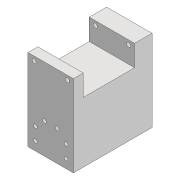
# Autodesk Inventor part: link
Saved by Autodesk Inventor 2020 (Build 240168000, 168)
## iProperties
Created: 2020-11-09
Part Number: link
Material: 일반
Document SubType Name: Modeling
Designer: 이호석
Mass: 68.2224 g
Surface Area: 145.151 cm^2
Volume: 68.2224 cm^3
Density: 1 g/cm^3
Appearance: 기본값
Author: 이호석
Autodesk Inventor part; units mm, degrees
ref_plane "YZ Plane" through (0, 0, 0) normal (1, 0, 0) x (0, 1, 0)
ref_plane "XZ Plane" through (0, 0, 0) normal (0, 1, 0) x (-1, 0, 0)
ref_plane "XY Plane" through (0, 0, 0) normal (0, 0, 1) x (1, 0, 0)
sketch "스케치1" plane through (0, 0, 0) normal (0, 0, 1) x (1, 0, 0)
  arc A0 (15, 100.5) -> (13, 102.5) centre (13, 100.5) ccw projected
  line L0 (13, 102.5) -> (-13, 102.5) projected
  arc A1 (-13, 102.5) -> (-15, 100.5) centre (-13, 100.5) ccw projected
  line L1 (-15, 100.5) -> (-15, -100.5) projected
  arc A2 (-15, -100.5) -> (-13, -102.5) centre (-13, -100.5) ccw projected
  line L2 (-13, -102.5) -> (-7, -102.5) projected
  arc A3 (-7, -102.5) -> (-5, -100.5) centre (-7, -100.5) ccw projected
  line L3 (-5, -100.5) -> (-5, -92.5) projected
  arc A4 (5, -92.5) -> (-5, -92.5) centre (0, -92.5) ccw projected
  line L4 (5, -92.5) -> (5, -100.5) projected
  arc A5 (5, -100.5) -> (7, -102.5) centre (7, -100.5) ccw projected
  line L5 (7, -102.5) -> (13, -102.5) projected
  arc A6 (13, -102.5) -> (15, -100.5) centre (13, -100.5) ccw projected
  line L6 (15, -100.5) -> (15, 100.5) projected
  circle A7 centre (7.7782, -100.2782) radius 1.25 projected
  circle A8 centre (0, -81.5) radius 1.25 projected
  circle A9 centre (-11, -92.5) radius 1.25 projected
  circle A10 centre (11, -92.5) radius 1.25 projected
  circle A11 centre (-7.7782, -100.2782) radius 1.25 projected
  circle A12 centre (7.7782, -84.7218) radius 1.25 projected
  circle A13 centre (-7.7782, -84.7218) radius 1.25 projected
  circle A14 centre (-10.1627, 76.7095) radius 1.25 projected
  circle A15 centre (-10.1627, 68.2905) radius 1.25 projected
  circle A16 centre (10.1627, 68.2905) radius 1.25 projected
  circle A17 centre (10.1627, 76.7095) radius 1.25 projected
  circle A18 centre (4.2095, 82.6627) radius 1.25 projected
  circle A19 centre (-4.2095, 82.6627) radius 1.25 projected
  line L7 (0, 102.5) -> (0, 82.5)
  line L8 (15, 102.5) -> (-15, 102.5)
  line L9 (-15, 102.5) -> (-15, 62.5)
  line L10 (-15, 62.5) -> (15, 62.5)
  line L11 (15, 62.5) -> (15, 102.5)
  line L12 (15, 102.5) -> (-15, 62.5) construction
  line L13 (-15, 102.5) -> (15, 62.5) construction
  point P0 (0, 0)
  dimension "d0" = 20
  dimension "d1" = 40
  constraints: 14 end point, 3 midpoint, 2 parallel, 1 horizontal, 1 perpendicular, 1 point on line, 1 vertical
  measures "d0" distance of L7.start L7.end
  measures "d1" distance of L9.end L8.end
ref_plane "작업 평면1" through (-15, -102.5, 52) normal (0, 0, -1) x (0, 1, 0)
extrude "돌출1" add sketch "스케치1" along normal up to surface (52 mm away) contours L6 L10 L1 A1 L0 A0
sketch "스케치2" plane through (-13, 102.5, 0) normal (0, 1, 0) x (1, 0, 0)
  line L0 (-0.4121, -11.5) -> (26.4121, -11.5) projected
  line L1 (-0.4121, -45.5) -> (26.4121, -45.5) projected
  line L2 (-2, 0) -> (-2, -52) projected
  line L3 (28, 0) -> (28, -52) projected
  line L4 (-2, -52) -> (28, -52)
  line L5 (28, -52) -> (28, -45.5)
  line L6 (28, -45.5) -> (-2, -45.5)
  line L7 (-2, -45.5) -> (-2, -52)
  line L8 (-2, 0) -> (28, 0)
  line L9 (28, 0) -> (28, -11.5)
  line L10 (28, -11.5) -> (-2, -11.5)
  line L11 (-2, -11.5) -> (-2, 0)
  point P0 (13, 0)
  dimension "d4" = 30
  constraints: 16 end point, 4 parallel, 3 point on line, 2 horizontal, 2 perpendicular
  measures "d4" distance of L9.end L10.end
ref_plane "작업 평면2" through (-7.15, 116.5, 9.5) normal (0, -1, 0) x (1, 0, 0)
extrude "돌출2" add sketch "스케치2" along normal up to surface (14 mm away) contours L10 L2 L8 L3 L0 | L6 L1 L3 L4 L2
sketch "스케치3" plane through (0, 0, 0) normal (0, 0, -1) x (-1, 0, 0)
  line L0 (-15, 102.5) -> (-13, 102.5) projected
  line L1 (-15, 62.5) -> (-15, 100.5) projected
  line L2 (-15, 102.5) -> (-15, 100.5)
  line L3 (15, 100.5) -> (15, 62.5) projected
  line L4 (-15, 100.5) -> (15, 100.5)
  line L5 (15, 100.5) -> (15, 102.5)
  arc A0 (15, 100.5) -> (13, 102.5) centre (13, 100.5) ccw projected
  line L6 (-15, 102.5) -> (15, 102.5)
  line L7 (13, 102.5) -> (-13, 102.5) projected
  point P0 (0, 0)
  constraints: 8 end point, 2 perpendicular, 1 collinear, 1 tangent, 1 vertical
extrude "돌출3" add sketch "스케치3" against normal up to surface (52 mm away)
sketch "스케치4" plane through (0, 0, 0) normal (0, 0, -1) x (-1, 0, 0)
  circle A0 centre (-17.3, 119) radius 1.35 projected
  circle A1 centre (17.3, 119) radius 1.35 projected
  line L0 (-20.1, 119.3234) -> (-20.1, 163.5766) projected
  arc A2 (-20.1, 119.3234) -> (-19.5808, 117.6364) centre (-17.1, 119.3234) ccw projected
  line L1 (-15.8929, 112.2131) -> (-19.5808, 117.6364) projected
  arc A3 (-15.8929, 112.2131) -> (-13.4121, 110.9) centre (-13.4121, 113.9) ccw projected
  line L2 (13.4121, 110.9) -> (-13.4121, 110.9) projected
  arc A4 (13.4121, 110.9) -> (15.8929, 112.2131) centre (13.4121, 113.9) ccw projected
  line L3 (19.5808, 117.6364) -> (15.8929, 112.2131) projected
  arc A5 (19.5808, 117.6364) -> (20.1, 119.3234) centre (17.1, 119.3234) ccw projected
  line L4 (20.1, 163.5766) -> (20.1, 119.3234) projected
  arc A6 (20.1, 163.5766) -> (19.5808, 165.2636) centre (17.1, 163.5766) ccw projected
  line L5 (15.5953, 171.1246) -> (19.5808, 165.2636) projected
  arc A7 (15.5953, 171.1246) -> (13.9414, 172) centre (13.9414, 170) ccw projected
  line L6 (6.65, 172) -> (13.9414, 172) projected
  arc A8 (8.15, 170.5) -> (6.65, 172) centre (6.65, 170.5) ccw projected
  line L7 (8.15, 170.5) -> (8.15, 168) projected
  arc A9 (8.15, 168) -> (10.5, 165.65) centre (10.5, 168) ccw projected
  line L8 (10.5, 165.65) -> (13.5, 165.65) projected
  arc A10 (14.5, 164.65) -> (13.5, 165.65) centre (13.5, 164.65) ccw projected
  line L9 (14.5, 164.65) -> (14.5, 123.85) projected
  arc A11 (13.5, 122.85) -> (14.5, 123.85) centre (13.5, 123.85) ccw projected
  line L10 (13.5, 122.85) -> (10.5, 122.85) projected
  arc A12 (10.5, 122.85) -> (8.15, 120.5) centre (10.5, 120.5) ccw projected
  line L11 (8.15, 120.5) -> (8.15, 117.5) projected
  arc A13 (7.15, 116.5) -> (8.15, 117.5) centre (7.15, 117.5) ccw projected
  line L12 (7.15, 116.5) -> (-7.15, 116.5) projected
  arc A14 (-8.15, 117.5) -> (-7.15, 116.5) centre (-7.15, 117.5) ccw projected
  line L13 (-8.15, 117.5) -> (-8.15, 120.5) projected
  arc A15 (-8.15, 120.5) -> (-10.5, 122.85) centre (-10.5, 120.5) ccw projected
  line L14 (-10.5, 122.85) -> (-13.5, 122.85) projected
  arc A16 (-14.5, 123.85) -> (-13.5, 122.85) centre (-13.5, 123.85) ccw projected
  line L15 (-14.5, 123.85) -> (-14.5, 164.65) projected
  arc A17 (-13.5, 165.65) -> (-14.5, 164.65) centre (-13.5, 164.65) ccw projected
  line L16 (-13.5, 165.65) -> (-10.5, 165.65) projected
  arc A18 (-10.5, 165.65) -> (-8.15, 168) centre (-10.5, 168) ccw projected
  line L17 (-8.15, 168) -> (-8.15, 170.5) projected
  arc A19 (-6.65, 172) -> (-8.15, 170.5) centre (-6.65, 170.5) ccw projected
  line L18 (-13.9414, 172) -> (-6.65, 172) projected
  arc A20 (-13.9414, 172) -> (-15.5953, 171.1246) centre (-13.9414, 170) ccw projected
  line L19 (-19.5808, 165.2636) -> (-15.5953, 171.1246) projected
  arc A21 (-19.5808, 165.2636) -> (-20.1, 163.5766) centre (-17.1, 163.5766) ccw projected
  arc A22 (15.95, 163) -> (18.65, 163) centre (17.3, 163) ccw projected
  arc A23 (18.65, 163) -> (15.95, 163) centre (17.3, 163) ccw projected
  arc A24 (15.95, 141) -> (18.65, 141) centre (17.3, 141) ccw projected
  arc A25 (18.65, 141) -> (15.95, 141) centre (17.3, 141) ccw projected
  arc A26 (9.65, 113.7) -> (12.35, 113.7) centre (11, 113.7) ccw projected
  arc A27 (12.35, 113.7) -> (9.65, 113.7) centre (11, 113.7) ccw projected
  arc A28 (-18.65, 163) -> (-15.95, 163) centre (-17.3, 163) ccw projected
  arc A29 (-15.95, 163) -> (-18.65, 163) centre (-17.3, 163) ccw projected
  arc A30 (-18.65, 141) -> (-15.95, 141) centre (-17.3, 141) ccw projected
  arc A31 (-15.95, 141) -> (-18.65, 141) centre (-17.3, 141) ccw projected
  arc A32 (-12.35, 113.7) -> (-9.65, 113.7) centre (-11, 113.7) ccw projected
  arc A33 (-9.65, 113.7) -> (-12.35, 113.7) centre (-11, 113.7) ccw projected
  point P0 (0, 0)
extrude "돌출4" cut sketch "스케치4" against normal through all contours A27 A26 | A33 A32
